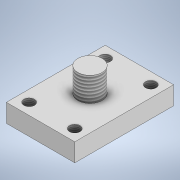
# Autodesk Inventor part: conector cardan
Saved by Autodesk Inventor 2021 (Build 250183000, 183)
## iProperties
Created: 2021-04-23
Part Number: conector cardan
Material: Genérico
Document SubType Name: Modeling
Designer: equip
Density: 1 g/cm^3
Appearance: Valor por defecto
Author: equip
Autodesk Inventor part; units mm, degrees
ref_plane "YZ Plane" through (0, 0, 0) normal (1, 0, 0) x (0, 1, 0)
ref_plane "XZ Plane" through (0, 0, 0) normal (0, 1, 0) x (-1, 0, 0)
ref_plane "XY Plane" through (0, 0, 0) normal (0, 0, 1) x (1, 0, 0)
sketch "Boceto1" plane through (0, 0, 0) normal (0, 1, 0) x (-1, 0, 0)
  circle A0 centre (0, 0) radius 8
  line L0 (0, 0) -> (0, 22.5) construction
  line L1 (0, 22.5) -> (-32.5, 22.5) construction
  line L2 (-32.5, 22.5) -> (32.5, 22.5)
  line L3 (32.5, 22.5) -> (32.5, -22.5)
  line L4 (32.5, -22.5) -> (-32.5, -22.5)
  line L5 (-32.5, -22.5) -> (-32.5, 22.5)
  dimension "d0" = 16
  dimension "d1" = 22.5
  dimension "d2" = 32.5
  dimension "d3" = 65
  dimension "d4" = 45
  constraints: 12 end point, 2 parallel, 2 perpendicular, 1 centre point, 1 coincident, 1 horizontal, 1 vertical
  measures "d0" diameter of A0
  measures "d1" distance of L0.start L0.end
  measures "d2" distance of L0.end L1.end
  measures "d3" distance of L3.end L4.end
  measures "d4" distance of L2.end L3.end
extrude "Extrusión1" add sketch "Boceto1" along normal blind 16 contours A0
sketch "Boceto2" plane through (0, 0, 0) normal (0, -1, 0) x (1, 0, 0)
  line L0 (0, 0) -> (-22.5, 0) construction
  line L1 (-22.5, 0) -> (-22.5, -32.5) construction
  line L2 (-22.5, -32.5) -> (22.5, -32.5)
  line L3 (22.5, -32.5) -> (22.5, 32.5)
  line L4 (22.5, 32.5) -> (-22.5, 32.5)
  line L5 (-22.5, 32.5) -> (-22.5, -32.5)
  dimension "d7" = 22.5
  dimension "d8" = 32.5
  dimension "d9" = 45
  dimension "d10" = 65
  constraints: 12 end point, 2 horizontal, 2 parallel, 2 perpendicular
  measures "d7" distance of L0.start L0.end
  measures "d8" distance of L0.end L1.end
  measures "d9" distance of L4.end L3.end
  measures "d10" distance of L3.end L2.end
extrude "Extrusión2" add sketch "Boceto2" along normal blind 12
thread "Rosca1" size "M16x2" class "6g" standard "ANSI Metric M Profile" full length
sketch "Boceto3" plane through (0, 0, 0) normal (0, 1, 0) x (1, 0, 0)
  line L0 (0, 0) -> (0, -25) construction
  line L1 (0, -25) -> (15, -25) construction
  line L2 (15, -25) -> (-15, -25) construction
  line L3 (-15, -25) -> (-15, 25) construction
  line L4 (-15, 25) -> (15, 25) construction
  line L5 (15, 25) -> (15, -25) construction
  circle A0 centre (-15, -25) radius 3.5
  circle A1 centre (15, -25) radius 3.5
  circle A2 centre (-15, 25) radius 3.5
  circle A3 centre (15, 25) radius 3.5
  dimension "d15" = 25
  dimension "d16" = 15
  dimension "d17" = 30
  dimension "d18" = 50
  dimension "d19" = 30
  dimension "d20" = 7
  dimension "d21" = 7
  dimension "d22" = 7
  dimension "d23" = 7
  constraints: 12 end point, 4 centre point, 4 coincident, 3 perpendicular, 1 point on line, 1 vertical
  measures "d15" distance of L0.start L0.end
  measures "d16" distance of L0.end L1.end
  measures "d17" distance of L1.end L2.end
  measures "d18" distance of L2.end L3.end
  measures "d19" distance of L3.end L4.end
  measures "d20" diameter of A0
  measures "d21" diameter of A1
  measures "d22" diameter of A2
  measures "d23" diameter of A3
extrude "Extrusión3" cut sketch "Boceto3" against normal blind 12
thread "Rosca2" size "M7x1" class "6H" standard "ANSI Metric M Profile" full length
thread "Rosca3" size "M7x1" class "6H" standard "ANSI Metric M Profile" full length
thread "Rosca4" size "M7x1" class "6H" standard "ANSI Metric M Profile" full length
thread "Rosca5" size "M7x1" class "6H" standard "ANSI Metric M Profile" full length
